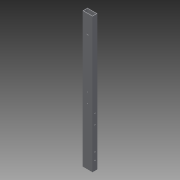
# Autodesk Inventor part: SuperSuperStructure
Saved by Autodesk Inventor 2013 (Build 170138000, 138)
## iProperties
Created: 2014-01-18
Part Number: SuperSuperStructure
Material: Generic
Document SubType Name: Modeling
Designer: 215152
Density: 1 g/cm^3
Author: 215152
Autodesk Inventor part; units mm, degrees
ref_plane "YZ Plane" through (0, 0, 0) normal (1, 0, 0) x (0, 1, 0)
ref_plane "XZ Plane" through (0, 0, 0) normal (0, 1, 0) x (-1, 0, 0)
ref_plane "XY Plane" through (0, 0, 0) normal (0, 0, 1) x (1, 0, 0)
sketch "Sketch1" plane through (0, 0, 0) normal (0, 1, 0) x (-1, 0, 0)
  line L0 (-25.4, -12.7) -> (25.4, -12.7)
  line L1 (25.4, -12.7) -> (25.4, 12.7)
  line L2 (25.4, 12.7) -> (-25.4, 12.7)
  line L3 (-25.4, 12.7) -> (-25.4, -12.7)
  line L4 (-25.4, -12.7) -> (25.4, 12.7) construction
  line L5 (25.4, -12.7) -> (-25.4, 12.7) construction
  line L6 (22.225, -9.525) -> (-22.225, -9.525)
  line L7 (-22.225, -9.525) -> (-22.225, 9.525)
  line L8 (-22.225, 9.525) -> (22.225, 9.525)
  line L9 (22.225, 9.525) -> (22.225, -9.525)
  line L10 (22.225, -9.525) -> (-22.225, 9.525) construction
  line L11 (-22.225, -9.525) -> (22.225, 9.525) construction
  point P0 (0, 0)
  dimension "d0" = 50.8
  dimension "d1" = 25.4
  dimension "d2" = 44.45
  dimension "d3" = 19.05
  constraints: 24 end point, 4 midpoint, 4 parallel, 2 horizontal, 2 perpendicular
  measures "d0" distance of L2.end L1.end
  measures "d1" distance of L1.end L0.end
  measures "d2" distance of L7.end L8.end
  measures "d3" distance of L6.end L7.end
extrude "Extrusion1" add sketch "Sketch1" along normal blind 609.6
sketch "Sketch2" plane through (-25.4, 0, 12.7) normal (0, 0, 1) x (1, 0, 0)
  line L0 (0, 609.6) -> (25.4, 609.6)
  line L1 (25.4, 609.6) -> (25.4, 584.2)
  line L2 (25.4, 584.2) -> (0, 584.2)
  line L3 (0, 584.2) -> (0, 609.6)
  circle A0 centre (25.4, 584.2) radius 6.35
  point P0 (25.4, 0)
  dimension "d6" = 25.4
  dimension "d7" = 25.4
  dimension "d8" = 12.7
  constraints: 8 end point, 2 parallel, 1 centre point, 1 coincident, 1 horizontal, 1 perpendicular
  measures "d6" distance of L1.end L2.end
  measures "d7" distance of L0.end L1.end
  measures "d8" diameter of A0
extrude "Extrusion2" cut sketch "Sketch2" against normal blind 609.6 contours A0 L2 L1 | L1 L2 A0
sketch "Sketch4" plane through (0, 0, 0) normal (0, -1, 0) x (1, 0, 0)
  line L0 (22.225, 9.525) -> (22.225, -9.525) projected
  line L1 (22.225, -9.525) -> (-22.225, -9.525) projected
  line L2 (-22.225, -9.525) -> (-22.225, 9.525) projected
  line L3 (-22.225, 9.525) -> (22.225, 9.525) projected
  line L4 (25.4, -12.7) -> (-25.4, -12.7) projected
  line L5 (25.4, 12.7) -> (25.4, -12.7) projected
  line L6 (-25.4, 12.7) -> (25.4, 12.7) projected
  line L7 (-25.4, -12.7) -> (-25.4, 12.7) projected
  point P0 (0, 0)
extrude "Extrusion4" add sketch "Sketch4" along normal blind 12.7
sketch "Sketch6" plane through (0, 609.6, 0) normal (0, 1, 0) x (1, 0, 0)
  line L0 (22.225, 9.525) -> (22.225, -9.525) projected
  line L1 (22.225, -9.525) -> (-22.225, -9.525) projected
  line L2 (-22.225, -9.525) -> (-22.225, 9.525) projected
  line L3 (-22.225, 9.525) -> (22.225, 9.525) projected
  line L4 (25.4, 12.7) -> (-25.4, 12.7) projected
  line L5 (-25.4, 12.7) -> (-25.4, -12.7) projected
  line L6 (-25.4, -12.7) -> (25.4, -12.7) projected
  line L7 (25.4, -12.7) -> (25.4, 12.7) projected
  point P0 (0, 0)
extrude "Extrusion6" add sketch "Sketch6" along normal blind 63.5
sketch "Sketch8" plane through (-25.4, -12.7, 12.7) normal (0, 0, 1) x (1, 0, 0)
  line L0 (50.8, 0) -> (50.8, 685.8) projected
  line L1 (0, 685.8) -> (50.8, 685.8) projected
  line L2 (25.4, 685.8) -> (25.4, 341.8078)
  line L3 (25.4, 685.8) -> (369.3922, 685.8) construction
  line L4 (25.4, 341.8078) -> (25.4, 291.0078)
  circle A0 centre (25.4, 291.0078) radius 3.175
  circle A1 centre (25.4, 341.8078) radius 3.175
  point P0 (25.4, 12.7)
  dimension "d49" = 343.9922
  dimension "d50" = 90
  dimension "d51" = 50.8
  dimension "d52" = 180
  dimension "d53" = 6.35
  dimension "d54" = 6.35
  constraints: 6 end point, 2 centre point, 2 coincident, 2 parallel, 1 horizontal, 1 midpoint, 1 perpendicular
  measures "d49" distance of L2.start L2.end
  measures "d50" angle of L2 L3
  measures "d51" distance of L2.end L4.end
  measures "d52" angle of L4 L2
  measures "d53" diameter of A0
  measures "d54" diameter of A1
extrude "Extrusion9" cut sketch "Sketch8" against normal blind 50.8
sketch "Sketch9" plane through (25.4, -12.7, 12.7) normal (1, 0, 0) x (0, 0, -1)
  line L0 (25.4, 0) -> (0, 0) projected
  line L1 (12.7, 0) -> (12.7, 84.1502)
  line L2 (12.7, 84.1502) -> (12.7, 46.0502)
  line L3 (12.7, 84.1502) -> (50.8, 84.1502) construction
  point P0 (12.7, 12.7)
  dimension "d57" = 84.1502
  dimension "d58" = 38.1
  dimension "d59" = 90
  constraints: 6 end point, 2 coincident, 2 perpendicular, 1 collinear, 1 horizontal, 1 midpoint
  measures "d57" distance of L1.start L1.end
  measures "d58" distance of L1.end L2.end
  measures "d59" angle of L2 L3
hole "Hole1" at (25.4, 71.4502, 0) at (25.4, 33.3502, 0) direction (-1, 0, 0) diameter 6.35 end through all
sketch "Sketch10" plane through (-25.4, -12.7, 12.7) normal (0, 0, 1) x (1, 0, 0)
  circle A0 centre (25.4, 341.8078) radius 3.175 projected
  circle A1 centre (25.4, 596.9) radius 6.35 projected
  line L0 (50.8, 0) -> (50.8, 685.8) projected
  line L1 (0, 0) -> (0, 685.8) projected
  line L2 (50.8, 0) -> (0, 0) projected
  line L3 (25.4, 341.8078) -> (25.4, 354.5078)
  line L4 (25.4, 341.8078) -> (38.1, 341.8078) construction
  line L5 (25.4, 354.5078) -> (50.8, 354.5078)
  line L6 (25.4, 354.5078) -> (0, 354.5078)
  line L7 (25.4, 596.9) -> (25.4, 501.65)
  line L8 (25.4, 501.65) -> (50.8, 501.65)
  line L9 (50.8, 501.65) -> (0, 501.65)
  line L10 (50.8, 501.65) -> (0, 501.65)
  line L11 (0, 501.65) -> (0, 354.5078)
  line L12 (0, 354.5078) -> (50.8, 354.5078)
  line L13 (50.8, 354.5078) -> (50.8, 501.65)
  line L14 (50.8, 501.65) -> (44.45, 501.65)
  line L15 (50.8, 495.3) -> (50.8, 501.65)
  line L16 (28.575, 545.0078) -> (28.575, 506.9078)
  line L17 (28.575, 506.9078) -> (22.225, 506.9078)
  line L18 (22.225, 545.0078) -> (15.875, 534.0093)
  line L19 (44.45, 488.95) -> (57.15, 488.95) construction
  line L20 (15.875, 534.0093) -> (22.225, 534.0093)
  line L21 (44.45, 476.25) -> (38.1, 476.25)
  line L22 (38.1, 494.2078) -> (38.1, 500.5578)
  line L23 (12.7, 500.5578) -> (12.7, 478.3328)
  line L24 (22.225, 476.25) -> (22.225, 469.9)
  line L25 (44.45, 469.9) -> (44.45, 476.25)
  line L26 (12.7, 476.25) -> (6.35, 476.25)
  line L27 (22.225, 476.25) -> (22.225, 469.9)
  line L28 (12.7, 462.4578) -> (12.7, 468.8078)
  line L29 (6.35, 469.9) -> (6.35, 476.25)
  line L30 (22.225, 476.25) -> (28.575, 476.25)
  line L31 (28.575, 456.1078) -> (22.225, 456.1078)
  arc A2 (38.1, 473.5703) -> (26.9875, 484.6828) centre (26.8738, 473.4566) ccw
  line L32 (17.4625, 450.85) -> (33.1779, 450.85) construction
  arc A3 (26.9875, 462.4578) -> (38.1, 473.5703) centre (26.8738, 473.684) ccw
  arc A4 (26.9875, 468.8078) -> (26.9875, 478.3328) centre (26.9875, 473.5703) ccw
  line L33 (6.35, 476.25) -> (12.7, 476.25)
  line L34 (28.575, 456.1078) -> (28.575, 418.0078)
  line L35 (28.575, 418.0078) -> (22.225, 418.0078)
  line L36 (22.225, 456.1078) -> (15.875, 445.1093)
  line L37 (44.45, 438.15) -> (57.15, 438.15) construction
  line L38 (15.875, 445.1093) -> (22.225, 445.1093)
  line L39 (44.45, 431.8) -> (6.35, 431.8)
  line L40 (44.45, 392.6078) -> (31.75, 405.3078) construction
  line L41 (44.45, 412.75) -> (62.4105, 412.75) construction
  line L42 (44.45, 392.6078) -> (31.75, 379.9078) construction
  line L43 (44.45, 412.75) -> (62.4105, 412.75) construction
  line L44 (-3.7211, 402.6789) -> (19.05, 379.9078) construction
  line L45 (-3.7211, 402.6789) -> (28.4821, 402.6789) construction
  line L46 (-3.7211, 402.6789) -> (8.9789, 415.3789) construction
  line L47 (-3.7211, 402.6789) -> (14.2394, 402.6789) construction
  line L48 (25.4, 405.3078) -> (31.75, 405.3078) construction
  line L49 (19.05, 386.2578) -> (19.05, 398.9578)
  line L50 (31.75, 398.9578) -> (31.75, 386.2578)
  line L51 (19.05, 398.9578) -> (31.75, 386.2578) construction
  line L52 (31.75, 398.9578) -> (19.05, 386.2578) construction
  line L53 (12.7, 392.6078) -> (-3.7211, 402.6789)
  line L54 (24.6062, 373.508) -> (24.6062, 379.9576)
  line L55 (26.1937, 379.9576) -> (26.1937, 373.508)
  line L56 (-1.7923, 402.0764) -> (12.7498, 391.8141) construction
  line L57 (12.7498, 393.4016) -> (0.1062, 399.8942) construction
  line L58 (24.6062, 411.7076) -> (24.6062, 405.258)
  line L59 (26.1937, 405.258) -> (26.1937, 411.7076)
  line L60 (44.4998, 393.4016) -> (38.0502, 391.8141) construction
  line L61 (38.0502, 393.4016) -> (44.4998, 391.8141) construction
  line L62 (22.225, 545.0078) -> (28.575, 545.0078)
  line L63 (12.7, 527.05) -> (12.7, 488.95)
  line L64 (12.7, 488.95) -> (6.35, 488.95)
  line L65 (22.225, 506.9078) -> (22.225, 534.0093)
  line L66 (6.35, 516.0515) -> (0, 516.0515)
  line L67 (0, 516.0515) -> (6.35, 527.05)
  line L68 (44.45, 450.85) -> (38.1, 450.85)
  line L69 (38.1, 494.2078) -> (19.05, 494.2078)
  line L70 (19.05, 494.2078) -> (19.05, 484.6828)
  line L71 (19.05, 484.6828) -> (26.9875, 484.6828)
  line L72 (26.9875, 468.8078) -> (12.7, 468.8078)
  line L73 (12.7, 476.25) -> (6.35, 476.25)
  line L74 (12.7, 462.4578) -> (26.9875, 462.4578)
  line L75 (26.9875, 478.3328) -> (12.7, 478.3328)
  line L76 (22.225, 476.25) -> (44.45, 476.25)
  line L77 (12.7, 500.5578) -> (38.1, 500.5578)
  line L78 (44.45, 438.15) -> (33.4515, 444.5)
  line L79 (33.4515, 444.5) -> (33.4515, 438.15)
  line L80 (22.225, 445.1093) -> (22.225, 418.0078)
  line L81 (6.35, 438.15) -> (6.35, 431.8)
  line L82 (6.35, 431.8) -> (44.45, 431.8)
  line L83 (44.45, 431.8) -> (44.45, 438.15)
  line L84 (12.7, 398.9578) -> (12.7, 386.2578)
  line L85 (38.1, 386.2578) -> (38.1, 398.9578)
  line L86 (31.75, 386.2578) -> (19.05, 386.2578)
  line L87 (19.05, 398.9578) -> (31.75, 398.9578)
  arc A5 (24.6062, 405.258) -> (19.05, 398.9578) centre (25.4, 398.9578) ccw
  arc A6 (31.75, 398.9578) -> (26.1937, 405.258) centre (25.4, 398.9578) ccw
  arc A7 (19.05, 386.2578) -> (24.6062, 379.9576) centre (25.4, 386.2578) ccw
  arc A8 (26.1937, 379.9576) -> (31.75, 386.2578) centre (25.4, 386.2578) ccw
  arc A9 (24.6062, 411.7076) -> (12.7, 398.9578) centre (25.3998, 399.0324) ccw
  arc A10 (38.1, 398.9578) -> (26.1937, 411.7076) centre (25.4002, 399.0324) ccw
  arc A11 (12.7, 386.2578) -> (24.6062, 373.508) centre (25.3998, 386.1832) ccw
  arc A12 (26.1937, 373.508) -> (38.1, 386.2578) centre (25.4002, 386.1832) ccw
  line L88 (0, 685.8) -> (50.8, 685.8) projected
  line L89 (25.4, 354.5078) -> (25.4, 372.4656)
  line L90 (25.4, 354.5078) -> (25.4, 418.0078)
  line L91 (25.4, 418.0078) -> (22.225, 418.0078)
  line L92 (25.4, 354.5078) -> (25.4, 462.4578)
  line L93 (25.4, 462.4578) -> (25.4, 500.5578)
  line L94 (25.4, 500.5578) -> (25.4, 506.9078)
  line L95 (25.4, 506.9078) -> (22.225, 506.9078)
  point P0 (25.4, 12.7)
  point P1 (25.4, 392.6078)
  point P2 (4.4894, 397.6434)
  point P3 (41.275, 392.6078)
  point P4 (19.05, 514.35)
  dimension "d67" = 12.7
  dimension "d68" = 90
  dimension "d69" = 95.25
  dimension "d75" = 6.35
  dimension "d76" = 240
  dimension "d95" = 38.1
  dimension "d96" = 6.35
  dimension "d97" = 12.7
  dimension "d98" = 240
  dimension "d103" = 135
  dimension "d105" = 135
  dimension "d107" = 45
  dimension "d109" = 45
  dimension "d114" = 12.7
  dimension "d115" = 12.7
  dimension "d118" = 1.5875
  dimension "d119" = 6.35
  dimension "d120" = 6.35
  dimension "d121" = 6.35
  dimension "d122" = 6.35
  dimension "d123" = 12.7
  dimension "d124" = 12.7
  dimension "d125" = 12.7
  dimension "d126" = 12.7
  dimension "d128" = 6.35
  dimension "d140" = 38.1
  dimension "d141" = 17.9578
  dimension "d142" = 6.35
  dimension "d143" = 63.5
  dimension "d144" = 3.175
  dimension "d145" = 6.3002
  dimension "d146" = 107.95
  dimension "d147" = 25.4
  dimension "d148" = 14.2875
  dimension "d149" = 24.3078
  dimension "d150" = 38.1
  dimension "d151" = 6.35
  dimension "d152" = 3.175
  constraints: 184 end point, 22 point on circle, 16 perpendicular, 13 horizontal, 11 centre point, 11 parallel, 8 point on line, 7 equal length, 5 midpoint, 2 tangent, 1 coincident, 1 collinear
  measures "d67" distance of L3.start L3.end
  measures "d68" angle of L4 L3
  measures "d69" distance of L7.start L7.end
  measures "d75" distance of L64.start L64.end
  measures "d95" distance of L34.start L34.end
  measures "d96" distance of L83.start L83.end
  measures "d97" distance of L78.start L78.end
  measures "d103" angle of L41 L40
  measures "d105" angle of L42 L43
  measures "d107" angle of L44 L45
  measures "d109" angle of L47 L46
  measures "d114" distance of L86.start L86.end
  measures "d115" distance of L49.end L50.start
  measures "d118" distance of L54.end L55.start
  measures "d119" radius of A5
  measures "d120" radius of A6
  measures "d121" radius of A7
  measures "d122" radius of A8
  measures "d123" radius of A9
  measures "d124" radius of A10
  measures "d125" radius of A11
  measures "d126" radius of A12
  measures "d128" distance of L79.start L79.end
  measures "d140" distance of L3.end point (25.4, 392.608)
  measures "d141" distance of L3.end L89.end
  measures "d142" distance between parallel lines of L34 L80
  measures "d143" distance of L3.end L90.end
  measures "d144" distance of L90.end L91.end
  measures "d145" distance from line of L35 L58.start
  measures "d146" distance of L3.end L92.end
  measures "d147" distance of L23.start L22.end
  measures "d148" distance of L72.start L28.end
  measures "d149" distance from line of L77 L73.start
  measures "d150" distance of L92.end L93.end
  measures "d151" distance of L93.end L94.end
  measures "d152" distance of L94.end L95.end
extrude "Extrusion10" [suppressed]
sketch "Sketch11" plane through (25.4, -12.7, 12.7) normal (1, 0, 0) x (0, 0, -1)
  line L0 (0, 685.8) -> (25.4, 685.8) projected
  line L1 (0, 0) -> (0, 685.8) projected
  line L2 (12.7, 685.8) -> (12.7, 254)
  line L3 (12.7, 685.8) -> (444.5, 685.8) construction
  line L4 (12.7, 254) -> (12.7, 203.2)
  circle A0 centre (12.7, 254) radius 3.175
  circle A1 centre (12.7, 203.2) radius 3.175
  point P0 (12.7, 12.7)
  dimension "d132" = 431.8
  dimension "d133" = 90
  dimension "d134" = 50.8
  dimension "d135" = 180
  dimension "d136" = 6.35
  dimension "d137" = 6.35
  constraints: 6 end point, 2 centre point, 2 coincident, 2 parallel, 1 horizontal, 1 midpoint, 1 perpendicular
  measures "d132" distance of L2.start L2.end
  measures "d133" angle of L2 L3
  measures "d134" distance of L2.end L4.end
  measures "d135" angle of L4 L2
  measures "d136" diameter of A0
  measures "d137" diameter of A1
extrude "Extrusion11" cut sketch "Sketch11" against normal blind 50.8
body "Solid1"
